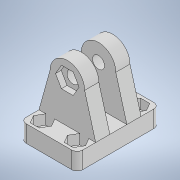
# Autodesk Inventor part: Support rotation
Saved by Autodesk Inventor 2022 (Build 260153000, 153)
## iProperties
Created: 2022-04-30
Part Number: Support rotation
Material: Générique
Document SubType Name: Modeling
Designer: victo
Density: 1 g/cm^3
Appearance: Par défaut
Author: victo
Autodesk Inventor part; units mm, degrees
ref_plane "YZ Plane" through (0, 0, 0) normal (1, 0, 0) x (0, 1, 0)
ref_plane "XZ Plane" through (0, 0, 0) normal (0, 1, 0) x (-1, 0, 0)
ref_plane "XY Plane" through (0, 0, 0) normal (0, 0, 1) x (1, 0, 0)
sketch "Vertical" plane through (0, 0, 0) normal (0, 0, 1) x (1, 0, 0)
  line L0 (10, -3) -> (-10, -3)
  line L1 (-10, -3) -> (-10, 3)
  line L2 (-10, 3) -> (10, 3)
  line L3 (10, 3) -> (10, -3)
  line L4 (10, -3) -> (-10, 3) construction
  line L5 (-10, -3) -> (10, 3) construction
  line L6 (-10, 3) -> (-6.1, 17)
  arc A0 (6.1, 17) -> (-6.1, 17) centre (0, 17) ccw
  line L7 (6.1, 17) -> (10, 3)
  line L8 (0, -8.22) -> (0, 28.32) projected
  circle A1 centre (0, 17) radius 2.1
  line L9 (-6.1, 17) -> (6.1, 17)
  circle A2 centre (0, 17) radius 4.1
  line L10 (-4.1569, 17) -> (-2.0785, 20.6)
  line L11 (-2.0785, 20.6) -> (2.0785, 20.6)
  line L12 (2.0785, 20.6) -> (4.1569, 17)
  line L13 (4.1569, 17) -> (2.0785, 13.4)
  line L14 (2.0785, 13.4) -> (-2.0785, 13.4)
  line L15 (-2.0785, 13.4) -> (-4.1569, 17)
  point P0 (0, 0)
  point P1 (0, 0)
  point P2 (-1.9621, 20.6)
  point P3 (-2.1366, 20.4993)
  point P4 (4.0988, 17.1007)
  point P5 (4.0988, 16.8993)
  point P6 (2.1366, 20.4993)
  point P7 (1.9621, 20.6)
  point P8 (1.9621, 13.4)
  point P9 (2.1366, 13.5007)
  point P10 (-2.1366, 13.5007)
  point P11 (-1.9621, 13.4)
  point P12 (-4.0988, 16.8993)
  point P13 (-4.0988, 17.1007)
  dimension "d6" = 6
  dimension "d7" = 20
  dimension "d8" = 14
  dimension "d9" = 4.2
  dimension "d10" = 4
  dimension "d11" = 8.2
  dimension "d12" = 20
  dimension "d34" = 7.2
  constraints: 30 end point, 4 midpoint, 3 centre point, 3 coincident, 3 point on line, 2 horizontal, 2 parallel, 2 point on circle, 1 equal length, 1 perpendicular, 13 other
  measures "d6" distance between parallel lines of L0 L2
  measures "d7" distance from line of L0 A0.centre
  measures "d8" distance from line of L2 A0.centre
  measures "d9" diameter of A1
  measures "d10" radial gap between concentric circles of A0 A1
  measures "d11" diameter of A2
  measures "d12" distance between parallel lines of L3 L1
  measures "d34" distance between parallel lines of L14 L11
extrude "Extrusion1" add sketch "Vertical" along normal mid plane 16 contours L2 L8 A2 L14 L13 L9 L7 | L2 L6 L9 L15 A2 L14 L8 | L9 L12 A2 L11 L8 A0 | A2 L14 L8 | L8 L14 A2 | L8 A2 L11 L10 L9 A0 | L13 A2 L9 | L9 A2 L12 | L14 A2 L15 L9 A1 L8 | L8 A1 L9 A2 L13 L14 | L14 L15 A2 | A2 L13 L14 | A2 L11 L8 | L8 L11 A2 | L9 A1 L8 L11 A2 L12 | L12 A2 | A2 L13 | L10 A2 L9 | L9 A2 L15 | A2 L15 | L8 A1 L9 A2 L10 L11 | L11 L12 A2 | A2 L10 L11 | A2 L10
extrude "Extrusion6" cut sketch "Vertical" against normal through all contours A2 L14 L8 | L8 L14 A2 | L14 A2 L15 L9 A1 L8 | L8 A1 L9 A2 L13 L14 | A2 L11 L8 | L8 L11 A2 | L9 A1 L8 L11 A2 L12 | L12 A2 | A2 L13 | A1 L9 L8 | L8 L9 A1 | A2 L15 | L8 A1 L9 A2 L10 L11 | L9 L8 A1 | A2 L10 | L9 A1 L8
extrude "Extrusion8" cut sketch "Vertical" along normal through all contours L13 A2 L9 | L9 A2 L12 | L14 A2 L15 L9 A1 L8 | L8 A1 L9 A2 L13 L14 | L14 L15 A2 | A2 L13 L14 | L9 A1 L8 L11 A2 L12 | L10 A2 L9 | L9 A2 L15 | A1 L9 L8 | L8 L9 A1 | L8 A1 L9 A2 L10 L11 | L11 L12 A2 | A2 L10 L11 | L9 L8 A1 | L9 A1 L8
extrude "Extrusion7" add sketch "Vertical" along normal mid plane 12 contours A2 L14 L8 | L8 L14 A2 | L13 A2 L9 | L9 A2 L12 | L14 A2 L15 L9 A1 L8 | L8 A1 L9 A2 L13 L14 | L14 L15 A2 | A2 L13 L14 | A2 L11 L8 | L8 L11 A2 | L9 A1 L8 L11 A2 L12 | L12 A2 | A2 L13 | L10 A2 L9 | L9 A2 L15 | A2 L15 | L8 A1 L9 A2 L10 L11 | L11 L12 A2 | A2 L10 L11 | A2 L10
extrude "Extrusion2" cut sketch "Vertical" along normal mid plane 6 contours L2 L8 A2 L14 L13 L9 L7 | L2 L6 L9 L15 A2 L14 L8 | L9 L12 A2 L11 L8 A0 | A2 L14 L8 | L8 L14 A2 | L8 A2 L11 L10 L9 A0 | L13 A2 L9 | L9 A2 L12 | L14 A2 L15 L9 A1 L8 | L8 A1 L9 A2 L13 L14 | L14 L15 A2 | A2 L13 L14 | A2 L11 L8 | L8 L11 A2 | L9 A1 L8 L11 A2 L12 | L12 A2 | A2 L13 | L10 A2 L9 | L9 A2 L15 | A1 L9 L8 | L8 L9 A1 | A2 L15 | L8 A1 L9 A2 L10 L11 | L11 L12 A2 | A2 L10 L11 | L9 L8 A1 | A2 L10 | L9 A1 L8
sketch "Horizontale" plane through (-10, 3, 8) normal (0, -1, 0) x (1, 0, 0)
  line L0 (0, -5) -> (20, -5) projected
  line L1 (20, -5) -> (20, 0) projected
  line L2 (0, 0) -> (20, 0) projected
  line L3 (0, -5) -> (0, 0) projected
  line L4 (20, -11) -> (0, -11) projected
  line L5 (0, -16) -> (0, -11) projected
  line L6 (20, -16) -> (0, -16) projected
  line L7 (20, -16) -> (20, -11) projected
  line L8 (20, -8) -> (0, -8) projected
  line L9 (0, -22.5) -> (20, -22.5)
  line L10 (20, -22.5) -> (20, 6.5)
  line L11 (20, 6.5) -> (0, 6.5)
  line L12 (0, 6.5) -> (0, -22.5)
  line L13 (0, -22.5) -> (20, 6.5) construction
  line L14 (20, -22.5) -> (0, 6.5) construction
  line L15 (4, -18.75) -> (16, -18.75) construction
  line L16 (16, -18.75) -> (16, 2.75) construction
  line L17 (16, 2.75) -> (4, 2.75) construction
  line L18 (4, 2.75) -> (4, -18.75) construction
  line L19 (4, -18.75) -> (16, 2.75) construction
  line L20 (16, -18.75) -> (4, 2.75) construction
  circle A0 centre (16, 2.75) radius 1.5
  circle A1 centre (4, 2.75) radius 1.5
  circle A2 centre (16, -18.75) radius 1.5
  circle A3 centre (4, -18.75) radius 1.5
  line L21 (14.4123, 0) -> (12.8246, 2.75)
  line L22 (12.8246, 2.75) -> (14.4123, 5.5)
  line L23 (14.4123, 5.5) -> (17.5877, 5.5)
  line L24 (17.5877, 5.5) -> (19.1754, 2.75)
  line L25 (19.1754, 2.75) -> (17.5877, 0)
  line L26 (17.5877, 0) -> (14.4123, 0)
  line L27 (2.4123, 0) -> (0.8246, 2.75)
  line L28 (0.8246, 2.75) -> (2.4123, 5.5)
  line L29 (2.4123, 5.5) -> (5.5877, 5.5)
  line L30 (5.5877, 5.5) -> (7.1754, 2.75)
  line L31 (7.1754, 2.75) -> (5.5877, 0)
  line L32 (5.5877, 0) -> (2.4123, 0)
  line L33 (5.5877, -16) -> (7.1754, -18.75)
  line L34 (7.1754, -18.75) -> (5.5877, -21.5)
  line L35 (5.5877, -21.5) -> (2.4123, -21.5)
  line L36 (2.4123, -21.5) -> (0.8246, -18.75)
  line L37 (0.8246, -18.75) -> (2.4123, -16)
  line L38 (2.4123, -16) -> (5.5877, -16)
  line L39 (17.5877, -16) -> (19.1754, -18.75)
  line L40 (19.1754, -18.75) -> (17.5877, -21.5)
  line L41 (17.5877, -21.5) -> (14.4123, -21.5)
  line L42 (14.4123, -21.5) -> (12.8246, -18.75)
  line L43 (12.8246, -18.75) -> (14.4123, -16)
  line L44 (14.4123, -16) -> (17.5877, -16)
  point P0 (10, -8)
  point P1 (16, 0)
  point P2 (4, 0)
  point P3 (4, -16)
  point P4 (16, -16)
  point P5 (2.4123, 0)
  point P6 (5.5877, 0)
  point P7 (2.4123, -16)
  point P8 (14.4123, 0)
  point P9 (17.5877, 0)
  dimension "d17" = 5.5
  dimension "d18" = 3
  dimension "d19" = 1
  dimension "d20" = 12
  dimension "d21" = 21.5
  dimension "d28" = 6
  constraints: 72 end point, 8 coincident, 8 midpoint, 4 centre point, 4 parallel, 4 point on line, 3 equal length, 3 equal radius, 2 collinear, 2 horizontal, 2 perpendicular, 52 other
  measures "d17" distance between parallel lines of L26 L23
  measures "d18" diameter of A0
  measures "d19" distance between parallel lines of L11 L23
  measures "d20" distance between parallel lines of L16 L18
  measures "d21" distance of L15.end L16.end
  measures "d28" distance between parallel lines of L4 L0
extrude "Extrusion3" add sketch "Horizontale" along normal blind 6 contours L3 L2 L1 L0 | L0 L10 L8 L12 | L12 L11 L10 L2 L25 L24 L23 L22 L21 L31 L30 L29 L28 L27 | L8 L10 L4 L12 | L27 L28 L29 L30 L31 L2 | L4 L7 L6 L5 | L2 L21 L22 L23 L24 L25 | L6 L37 L36 L35 L34 L33 L43 L42 L41 L40 L39 L10 L9 L12 | L6 L33 L34 L35 L36 L37 | L39 L40 L41 L42 L43 L6 | A0 | A1 | A2 | A3
extrude "Extrusion4" cut sketch "Horizontale" along normal through all contours A0 | A1 | A2 | A3
extrude "Extrusion5" cut sketch "Horizontale" along normal blind 3.5 contours L27 L28 L29 L30 L31 L2 | L2 L21 L22 L23 L24 L25 | L6 L33 L34 L35 L36 L37 | L39 L40 L41 L42 L43 L6
fillet "Congé1" radius 2 4 edges at (10, 0, 14.5) (-10, 0, 14.5) (10, 0, -14.5) (-10, 0, -14.5)
